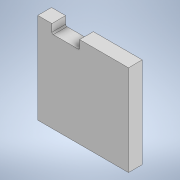
# Autodesk Inventor part: pcbOutline
Saved by Autodesk Inventor 2022 (Build 260153000, 153)
## iProperties
Created: 2023-11-22
Part Number: pcbOutline
Material: Generisch
Document SubType Name: Modeling
Designer: Marc Panse
Density: 1 g/cm^3
Appearance: Vorgabe
Author: Marc Panse
Autodesk Inventor part; units mm, degrees
ref_plane "YZ Plane" through (0, 0, 0) normal (1, 0, 0) x (0, 1, 0)
ref_plane "XZ Plane" through (0, 0, 0) normal (0, 1, 0) x (-1, 0, 0)
ref_plane "XY Plane" through (0, 0, 0) normal (0, 0, 1) x (1, 0, 0)
sketch "Skizze1" plane through (0, 0, 0) normal (0, 0, 1) x (1, 0, 0)
  line L0 (-33.02, -33.02) -> (33.02, -33.02)
  line L1 (33.02, -33.02) -> (33.02, 33.02)
  line L2 (33.02, 33.02) -> (-33.02, 33.02)
  line L3 (-33.02, 33.02) -> (-33.02, -33.02)
  line L4 (-33.02, -33.02) -> (33.02, 33.02) construction
  line L5 (33.02, -33.02) -> (-33.02, 33.02) construction
  line L6 (33.02, 33.02) -> (-2.54, 33.02)
  line L7 (-2.54, 33.02) -> (-22.733, 33.02)
  line L8 (-22.733, 33.02) -> (-2.54, 33.02)
  line L9 (-2.54, 33.02) -> (-2.54, 26.543)
  line L10 (-2.54, 26.543) -> (-22.733, 26.543)
  line L11 (-22.733, 26.543) -> (-22.733, 33.02)
  point P0 (0, 0)
  dimension "d0" = 66.04
  dimension "d1" = 66.04
  dimension "d2" = 35.56
  dimension "d3" = 20.193
  dimension "d4" = 6.477
  constraints: 24 end point, 4 parallel, 2 horizontal, 2 midpoint, 2 perpendicular, 2 point on line
  measures "d0" distance of L2.end L1.end
  measures "d1" distance between parallel lines of L0 L2
  measures "d2" distance of L1.end L6.end
  measures "d3" distance of L6.end L7.end
  measures "d4" distance of L8.end L9.end
extrude "Extrusion1" add sketch "Skizze1" along normal blind 10 contours L3 L2 L11 L10 L9 L1 L0
fillet "Rundung1" radius 1 2 edges at (-22.733, 26.543, 5) (-2.54, 26.543, 5)
